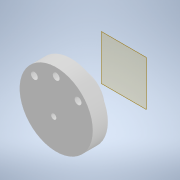
# Autodesk Inventor part: wheel_fixator_mirror
Saved by Autodesk Inventor 2022 (Build 260153000, 153)
## iProperties
Created: 2024-09-10
Part Number: wheel_fixator_mirror
Material: Типовые
Document SubType Name: Modeling
Designer: Andrey
Density: 1 g/cm^3
Appearance: По умолчанию
Author: Andrey
Autodesk Inventor part; units mm, degrees
ref_plane "YZ Plane" through (0, 0, 0) normal (1, 0, 0) x (0, 1, 0)
ref_plane "XZ Plane" through (0, 0, 0) normal (0, 1, 0) x (-1, 0, 0)
ref_plane "XY Plane" through (0, 0, 0) normal (0, 0, 1) x (1, 0, 0)
sketch "Эскиз1" plane through (0, 0, 0) normal (0, 0, 1) x (1, 0, 0)
  circle A0 centre (0, 0) radius 22.5
  dimension "d0" = 45
  constraints: 1 centre point, 1 coincident
  measures "d0" diameter of A0
extrude "Выдавливание1" add sketch "Эскиз1" along normal blind 9.295
sketch "Эскиз2" plane through (0, 0, 9.295) normal (0, 0, 1) x (1, 0, 0)
  circle A0 centre (0, 0) radius 12.6
  dimension "d3" = 25.2
  constraints: 1 centre point, 1 coincident
  measures "d3" diameter of A0
extrude "Выдавливание2" add sketch "Эскиз2" along normal blind 7.8
sketch "Эскиз3" plane through (0, 0, 9.295) normal (0, 0, 1) x (1, 0, 0)
  circle A0 centre (0, 0) radius 12.6 projected
  circle A1 centre (0, 0) radius 22.5 projected
  circle A2 centre (0, 0) radius 14.6
  dimension "d6" = 2
  constraints: 1 centre point
  measures "d6" radial gap between concentric circles of A0 A2
extrude "Выдавливание3" add sketch "Эскиз3" along normal blind 1 contours A2
chamfer "Фаска1" distance 0.5 angle 45 1 edges at (-14.6, 0, 10.295)
sketch "Эскиз4" plane through (0, 0, 17.095) normal (0, 0, 1) x (1, 0, 0)
  line L0 (0, 0) -> (0, 4)
  line L1 (0, 4) -> (3.4641, 2)
  line L2 (3.4641, 2) -> (3.4641, -2)
  line L3 (3.4641, -2) -> (0, -4)
  line L4 (0, -4) -> (-3.4641, -2)
  line L5 (-3.4641, -2) -> (-3.4641, 2)
  line L6 (-3.4641, 2) -> (0, 4)
  line L7 (3.9641, 2.2887) -> (0, 4.5774)
  line L8 (0, 4.5774) -> (-3.9641, 2.2887)
  line L9 (-3.9641, 2.2887) -> (-3.9641, -2.2887)
  line L10 (-3.9641, -2.2887) -> (0, -4.5774)
  line L11 (0, -4.5774) -> (3.9641, -2.2887)
  line L12 (3.9641, -2.2887) -> (3.9641, 2.2887)
  dimension "d12" = 4
  dimension "d13" = 0.5
  constraints: 26 end point, 1 coincident, 1 vertical, 18 other
  measures "d12" distance of L0.start L0.end
  measures "d13" distance between parallel lines of L1 L7
extrude "Выдавливание4" cut sketch "Эскиз4" against normal blind 7.8 contours L1 L2 L3 L4 L5 L6 | L12 L11 L10 L9 L8 L7
sketch "Эскиз5" plane through (0, 0, 0) normal (0, 0, -1) x (-1, 0, 0)
  circle A0 centre (13.4441, 11.2809) radius 1.5 projected
  circle A1 centre (0, 17.55) radius 1.5 projected
  circle A2 centre (-13.4441, 11.2809) radius 1.5 projected
  circle A3 centre (13.4441, 11.2809) radius 2.1
  circle A4 centre (0, 17.55) radius 2.1
  circle A5 centre (-13.4441, 11.2809) radius 2.1
  point P0 (0, 0)
  dimension "d16" = 4.2
  dimension "d17" = 4.2
  dimension "d18" = 4.2
  constraints: 3 centre point, 3 coincident
  measures "d16" diameter of A3
  measures "d17" diameter of A4
  measures "d18" diameter of A5
extrude "Выдавливание5" cut sketch "Эскиз5" against normal blind 7.8 contours A0 | A1 | A2 | A3 | A4 | A5
sketch "Эскиз6" plane through (0, 0, 17.095) normal (0, 0, 1) x (1, 0, 0)
  circle A0 centre (-1.5, -4.5) radius 1.5 projected
  circle A1 centre (-1.5, -4.5) radius 3.5
  point P0 (0, 0)
  dimension "d21" = 7
  constraints: 1 centre point, 1 coincident
  measures "d21" diameter of A1
extrude "Выдавливание6" cut sketch "Эскиз6" against normal blind 13 contours A0 | A1
sketch "Эскиз7" plane through (-1.5, -4.5, 4.095) normal (0, 0, 1) x (1, 0, 0)
  circle A0 centre (0, 0) radius 3.5 projected
  circle A1 centre (0, 0) radius 1.6
  point P0 (1.5, 4.5)
  dimension "d24" = 3.2
  constraints: 1 centre point, 1 coincident
  measures "d24" diameter of A1
extrude "Выдавливание7" cut sketch "Эскиз7" against normal blind 13 contours A1
ref_plane "РабПлоскость1" through (0, 0, 41.595) normal (0, 0, 1) x (1, 0, 0)
mirror "Зеркальное отражение1" about plane through (0, 0, 41.595) normal (0, 0, 1)
sketch "Эскиз8" plane through (0, 0, 0) normal (0, 0, -1) x (-1, 0, 0)
  circle A0 centre (0, 0) radius 38.8283
  constraints: 1 centre point, 1 coincident
extrude "Выдавливание8" cut sketch "Эскиз8" against normal blind 20
